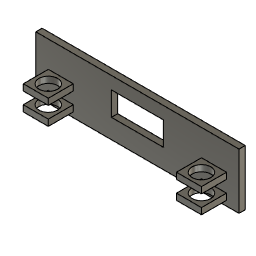
espmount (Autodesk Fusion 360 design; units mm, degrees)
Autodesk Fusion 360 part; units mm, degrees
sketch "Sketch1" plane through (0, 0, 0) normal (0, 1, 0) x (1, 0, 0)
  line L0 (2, -3.5) -> (30.5, -3.5)
  line L1 (30.5, -3.5) -> (30.5, -2)
  line L2 (30.5, -2) -> (2, -2)
  line L3 (2, -2) -> (2, -3.5)
  line L4 (12.5, -3.5) -> (20, -3.5)
  line L5 (20, -3.5) -> (20, -6.5)
  line L6 (20, -6.5) -> (12.5, -6.5)
  line L7 (12.5, -6.5) -> (12.5, -3.5)
  line L8 (12.1, -6.9) -> (20.4, -6.9)
  line L9 (20.4, -6.9) -> (20.4, -3.1)
  line L10 (20.4, -3.1) -> (12.1, -3.1)
  line L11 (12.1, -3.1) -> (12.1, -6.9)
  line L12 (0, -8.9) -> (32.5, -8.9)
  line L13 (32.5, -8.9) -> (32.5, 0)
  line L14 (32.5, 0) -> (0, 0)
  line L15 (0, 0) -> (0, -8.9)
  line L16 (30.5, -3.7) -> (26.5, -3.7)
  line L17 (26.5, -3.7) -> (26.5, -4.7)
  line L18 (26.5, -4.7) -> (30.5, -4.7)
  line L19 (30.5, -4.7) -> (30.5, -3.7)
  line L20 (26.5, -1.8) -> (30.5, -1.8)
  line L21 (30.5, -1.8) -> (30.5, -0.8)
  line L22 (30.5, -0.8) -> (26.5, -0.8)
  line L23 (26.5, -0.8) -> (26.5, -1.8)
  line L24 (2, -4.7) -> (6, -4.7)
  line L25 (6, -4.7) -> (6, -3.7)
  line L26 (6, -3.7) -> (2, -3.7)
  line L27 (2, -3.7) -> (2, -4.7)
  line L28 (2, -1.8) -> (6, -1.8)
  line L29 (6, -1.8) -> (6, -0.8)
  line L30 (6, -0.8) -> (2, -0.8)
  line L31 (2, -0.8) -> (2, -1.8)
  dimension "d1" = 28.5
  dimension "d2" = 1.5
  dimension "d3" = 7.5
  dimension "d4" = 3
  dimension "d5" = 10.5
  dimension "d6" = 0.4
  dimension "d7" = 0.4
  dimension "d8" = 0.4
  dimension "d9" = 0.4
  dimension "d10" = 2
  dimension "d11" = 2
  dimension "d12" = 2
  dimension "d13" = 2
  dimension "d30" = 4
  dimension "d31" = 1
  dimension "d32" = 0.2
  dimension "d33" = 4
  dimension "d34" = 4
  dimension "d35" = 1
  dimension "d36" = 0.2
  dimension "d37" = 4
  dimension "d38" = 4
  dimension "d39" = 1
  dimension "d40" = 4
  dimension "d41" = 1
  dimension "d42" = 4
  dimension "d43" = 4
  dimension "d44" = 0.2
  dimension "d45" = 0.2
  constraint horizontal L0
  constraint vertical L1
  constraint horizontal L2
  constraint vertical L3
  constraint horizontal L4
  constraint vertical L5
  constraint horizontal L6
  constraint vertical L7
  constraint coincident L0 L4.start
  constraint horizontal L8
  constraint vertical L9
  constraint horizontal L10
  constraint vertical L11
  constraint horizontal L12
  constraint vertical L13
  constraint horizontal L14
  constraint vertical L15
  constraint horizontal L16
  constraint vertical L17
  constraint horizontal L18
  constraint vertical L19
  constraint horizontal L20
  constraint vertical L21
  constraint horizontal L22
  constraint vertical L23
  constraint horizontal L24
  constraint vertical L25
  constraint horizontal L26
  constraint vertical L27
  constraint horizontal L28
  constraint vertical L29
  constraint horizontal L30
  constraint vertical L31
  constraint coincident L14.end L15.start
  measures "d1" distance of L0.start L0.end
  measures "d2" distance of L0.start L2.end
  measures "d3" distance of L4.start L4.end
  measures "d4" distance of L4.start L6.end
  measures "d5" distance of L3 L7
  measures "d6" distance of L5 L9
  measures "d7" distance of L7 L11
  measures "d8" distance of L6 L8
  measures "d9" distance of L0 L10
  measures "d10" distance of L8 L12
  measures "d11" distance of L2 L14
  measures "d12" distance of L1 L13
  measures "d13" distance of L3 L15
  measures "d30" distance of L16.start L16.end
  measures "d31" distance of L16.start L18.end
  measures "d32" distance of L0 L16
  measures "d33" distance of L1 L17
  measures "d34" distance of L20.start L20.end
  measures "d35" distance of L20.start L22.end
  measures "d36" distance of L2 L20
  measures "d37" distance of L1 L23
  measures "d38" distance of L24.start L24.end
  measures "d39" distance of L24.start L26.end
  measures "d40" distance of L28.start L28.end
  measures "d41" distance of L28.start L30.end
  measures "d42" distance of L3 L29
  measures "d43" distance of L3 L25
  measures "d44" distance of L0 L26
  measures "d45" distance of L2 L28
extrude "Extrude1" add sketch "Sketch1" along normal blind 2 contours L0 L1 L2 L3 L9 L10 L11 | L12 L13 L14 L15 | L16 L17 L18 L19 | L20 L21 L22 L23 | L24 L25 L26 L27 | L28 L29 L30 L31
extrude "Extrude4" cut 1 faces at (28.4667, 2, 4.1333) along direction (0, -1, 0) blind 1
extrude "Extrude5" add sketch "Sketch1" against normal blind 4 contours L16 L17 L18 L19 | L20 L21 L22 L23 | L24 L25 L26 L27 | L28 L29 L30 L31
sketch "Sketch3" plane through (0, 0, 4.7) normal (0, 0, 1) x (-1, 0, 0)
  line L0 (-6, 0) -> (-2, 0)
  line L1 (-2, 0) -> (-2, 4)
  line L2 (-2, 4) -> (-6, 4)
  line L3 (-6, 4) -> (-6, 0)
  circle A0 centre (-4, 2) radius 1.5
  circle A1 centre (-28.5, 2) radius 1.5
  dimension "d50" = 3
  dimension "d51" = 3
  measures "d50" diameter of A0
  measures "d51" diameter of A1
extrude "Extrude6" cut sketch "Sketch3" against normal blind 8 contours A0 | A1
equation "d5 = ( 21 / 2 ) * 1 mm"
